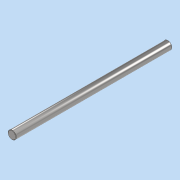
# Autodesk Inventor part: motorshaft2x38
Saved by Autodesk Inventor 2022 (Build 260153000, 153)
## iProperties
Created: 2024-04-30
Part Number: motorshaft2x38
Material: 鋼、合金
Document SubType Name: Modeling
Designer: ktamu
Density: 7.73 g/cm^3
Appearance: 半つや出し
Author: ktamu
Autodesk Inventor part; units mm, degrees
ref_plane "YZ Plane" through (0, 0, 0) normal (1, 0, 0) x (0, 1, 0)
ref_plane "XZ Plane" through (0, 0, 0) normal (0, 1, 0) x (-1, 0, 0)
ref_plane "XY Plane" through (0, 0, 0) normal (0, 0, 1) x (1, 0, 0)
sketch "スケッチ1" plane through (0, 0, 0) normal (0, 0, 1) x (1, 0, 0)
  circle A0 centre (0, 0) radius 1
  dimension "d0" = 2
  constraints: 1 centre point, 1 coincident
  measures "d0" diameter of A0
extrude "押し出し1" add sketch "スケッチ1" along normal blind 38
chamfer "面取り1" distance 0.09 angle 45 1 edges at (-1, 0, 0)
chamfer "面取り2" distance 0.09 angle 45 1 edges at (-1, 0, 38)
